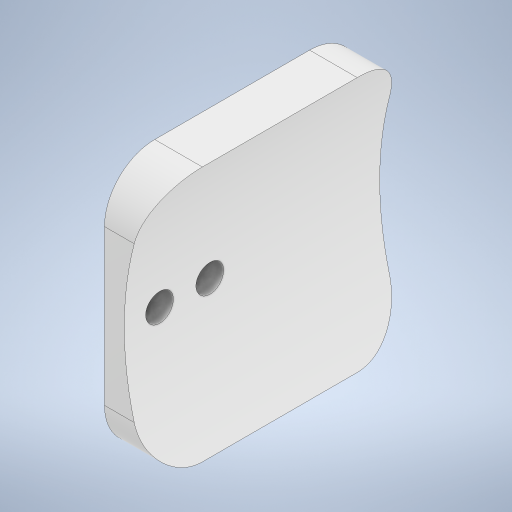
# Autodesk Inventor part: Pipe Holder
Saved by Autodesk Inventor 2023 (Build 270158030, 158C)
## iProperties
Created: 2022-10-01
Part Number: Pipe Holder
Material: ABS Plastic
Document SubType Name: Modeling
Designer: cjj5381
Density: 1.06 g/cm^3
Appearance: Smooth - White
Author: cjj5381
Autodesk Inventor part; units mm, degrees
ref_plane "YZ Plane" through (0, 0, 0) normal (1, 0, 0) x (0, 1, 0)
ref_plane "XZ Plane" through (0, 0, 0) normal (0, 1, 0) x (-1, 0, 0)
ref_plane "XY Plane" through (0, 0, 0) normal (0, 0, 1) x (1, 0, 0)
sketch "Sketch1" plane through (0, 0, 0) normal (0, 0, 1) x (1, 0, 0)
  line L0 (0, -25.4) -> (9.472, -25.4)
  line L1 (9.472, 25.4) -> (0, 25.4)
  line L2 (0, 25.4) -> (0, -25.4)
  circle A0 centre (65, 0) radius 61.0616 construction
  line L3 (0, 0) -> (-12.014, 0)
  arc A1 (9.472, 25.4) -> (9.472, -25.4) centre (65, 0) ccw
  point P0 (0, 0)
  dimension "d0" = 122.1232
  dimension "d1" = 65
  dimension "d2" = 50.8
  constraints: 8 end point, 2 horizontal, 2 midpoint, 2 point on circle, 1 centre point, 1 horizontal alignment, 1 parallel, 1 symmetric about line, 5 other
  measures "d1" distance of L3.start point (65, 0)
  measures "d2" distance of L1.end L0.start
extrude "Extrusion1" add sketch "Sketch1" along normal mid plane 50.8
sketch "Sketch2" plane through (0, -25.4, 25.4) normal (-1, 0, 0) x (0, 0, 1)
  circle A0 centre (-7, 25.4) radius 2.75
  circle A1 centre (-17, 25.4) radius 2.75
  line L0 (0, 50.8) -> (0, 0) projected
  point P0 (-25.4, 25.4)
  dimension "d8" = 5.5
  dimension "d9" = 7
  dimension "d10" = 10
  constraints: 2 centre point, 1 equal radius
  measures "d8" diameter of A0
  measures "d9" distance from line of L0 A0.centre
  measures "d10" distance of A0.centre A1.centre
extrude "Extrusion2" cut sketch "Sketch2" against normal through all
fillet "Fillet1" radius 10 4 edges at (4.736, 25.4, 25.4) (4.736, -25.4, 25.4) (4.736, 25.4, -25.4) (4.736, -25.4, -25.4)
body "Solid1"
